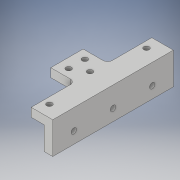
# Autodesk Inventor part: landingGearBracket
Saved by Autodesk Inventor 2018 (Build 220112000, 112)
## iProperties
Created: 2020-01-28
Part Number: landingGearBracket
Material: Generic
Document SubType Name: Modeling
Designer: anirudh.bali
Density: 1 g/cm^3
Appearance: Default
Author: anirudh.bali
Autodesk Inventor part; units mm, degrees
ref_plane "YZ Plane" through (0, 0, 0) normal (1, 0, 0) x (0, 1, 0)
ref_plane "XZ Plane" through (0, 0, 0) normal (0, 1, 0) x (-1, 0, 0)
ref_plane "XY Plane" through (0, 0, 0) normal (0, 0, 1) x (1, 0, 0)
sketch "Sketch1" plane through (0, 0, 0) normal (0, 1, 0) x (-1, 0, 0)
  line L0 (-0.9299, 13.6525) -> (-0.9299, 39.0525)
  line L1 (-0.9299, 13.6525) -> (-0.9299, 39.0525)
  line L2 (-0.9299, -13.6525) -> (-0.9299, -39.0525)
  arc A0 (-0.9299, 13.6525) -> (2.2451, 10.4775) centre (2.2451, 13.6525) ccw
  arc A1 (-0.9299, 13.6525) -> (2.2451, 10.4775) centre (2.2451, 13.6525) ccw
  arc A2 (2.2451, -10.4775) -> (-0.9299, -13.6525) centre (2.2451, -13.6525) ccw
  arc A3 (2.2451, -10.4775) -> (-0.9299, -13.6525) centre (2.2451, -13.6525) ccw
  line L3 (2.2451, 10.4775) -> (14.9451, 10.4775)
  line L4 (14.9451, 10.4775) -> (14.9451, -10.4775)
  line L5 (14.9451, -10.4775) -> (2.2451, -10.4775)
  line L6 (-9.3119, 39.0525) -> (-0.9299, 39.0525)
  line L7 (-9.3119, -39.0525) -> (-0.9299, -39.0525)
  line L8 (14.9451, 10.4775) -> (14.9451, -10.4775)
  circle A4 centre (8.5951, 5.2388) radius 1.75
  circle A5 centre (8.5951, -5.2388) radius 1.75
  circle A6 centre (0, 0) radius 1.75
  line L9 (-9.3119, 39.0525) -> (-9.3119, -39.0525)
  circle A7 centre (-5.1209, 31.4325) radius 1.75
  circle A8 centre (-5.1209, -31.4325) radius 1.75
  constraints: 20 end point, 9 centre point, 8 point on circle, 2 coincident, 2 perpendicular, 1 tangent
extrude "Extrusion1" add sketch "Sketch1" along normal blind 5.588
sketch "Sketch3" plane through (0, 5.588, 0) normal (0, 1, 0) x (1, 0, 0)
  line L0 (9.3119, -39.0525) -> (9.3119, 39.0525) projected
  line L1 (9.3119, -39.0525) -> (14.8999, -39.0525)
  line L2 (14.8999, -39.0525) -> (14.8999, 39.0525)
  line L3 (14.8999, 39.0525) -> (9.3119, 39.0525)
  line L4 (9.3119, 39.0525) -> (9.3119, -39.0525)
  point P0 (0, 0)
  dimension "d2" = 5.588
  constraints: 8 end point, 2 parallel, 1 horizontal, 1 perpendicular
  measures "d2" distance of L3.end L2.end
extrude "Extrusion2" add sketch "Sketch3" against normal blind 20.5994
sketch "Sketch4" plane through (14.8999, 5.588, 39.0525) normal (1, 0, 0) x (0, 0, -1)
  line L0 (0, -5.588) -> (0, 0) projected
  line L1 (49.53, 0) -> (28.575, 0) projected
  line L2 (0, -20.5994) -> (78.105, -20.5994) projected
  circle A0 centre (13.6525, -13.0937) radius 1.75
  circle A1 centre (39.0525, -13.0937) radius 1.75
  circle A2 centre (64.4525, -13.0937) radius 1.75
  point P0 (39.0525, -5.588)
  point P1 (78.105, 0)
  dimension "d8" = 3.5
  dimension "d9" = 3.5
  dimension "d10" = 3.5
  constraints: 3 centre point
  measures "d8" diameter of A0
  measures "d9" diameter of A1
  measures "d10" diameter of A2
extrude "Extrusion3" cut sketch "Sketch4" against normal blind 20.5994
body "Solid1"
